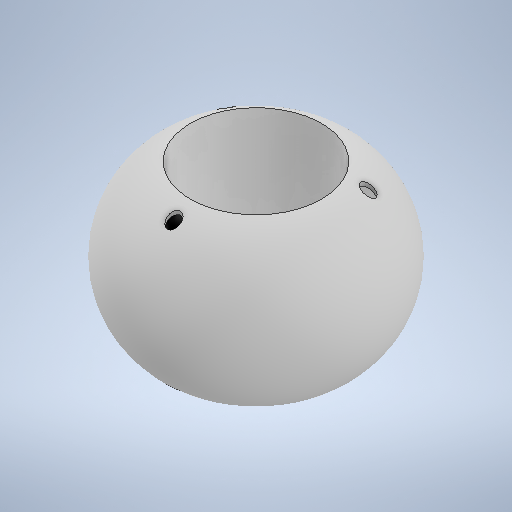
# Autodesk Inventor part: Buoy 5 HalfSphere
Saved by Autodesk Inventor 2025 (Build 290162000, 162)
## iProperties
Created: 2024-06-27
Part Number: Buoy 5 HalfSphere
Material: Generic
Document SubType Name: Modeling
Designer: track
Density: 1 g/cm^3
Appearance: Default
Author: track
Autodesk Inventor part; units mm, degrees
ref_plane "YZ Plane" through (0, 0, 0) normal (1, 0, 0) x (0, 1, 0)
ref_plane "XZ Plane" through (0, 0, 0) normal (0, 1, 0) x (-1, 0, 0)
ref_plane "XY Plane" through (0, 0, 0) normal (0, 0, 1) x (1, 0, 0)
sketch "Sketch1" plane through (0, 0, 0) normal (0, 0, 1) x (1, 0, 0)
  line L0 (0, 0) -> (0, 25.4) construction
  line L1 (30.48, 0) -> (30.48, 76.2)
  line L2 (0, 0) -> (30.48, 0)
  arc A0 (30.48, 0) -> (30.48, 76.2) centre (13.335, 38.1) ccw
  line L3 (31.98, 73.8048) -> (31.98, 2.3952)
  arc A1 (31.98, 2.3952) -> (31.98, 73.8048) centre (13.335, 38.1) ccw
  dimension "d0" = 25.4
  dimension "d1" = 30.48
  dimension "d2" = 76.2
  dimension "d8" = 17.145
  dimension "d9" = 1.5
  constraints: 8 end point, 4 point on circle, 2 centre point, 2 vertical, 1 horizontal, 1 other
  measures "d0" distance of L0.start L0.end
  measures "d1" distance between parallel lines of L1 L0
  measures "d2" distance of L1.start L1.end
  measures "d8" distance from line of A0.centre L1
  measures "d9" radial gap between concentric circles of A0 A1
revolve "Revolution1" add sketch "Sketch1" angle 360 about axis through (0, 0, 0) along (0, 1, 0)
sketch "Sketch2" plane through (0, 0, 0) normal (0, 1, 0) x (-1, 0, 0)
  circle A0 centre (0, 38.1) radius 3
  line L0 (0, 0) -> (0, 38.1) construction
  dimension "d11" = 6
  dimension "d12" = 38.1
  constraints: 2 end point, 1 centre point, 1 vertical
  measures "d11" diameter of A0
  measures "d12" distance of L0.start L0.end
extrude "Extrusion1" cut sketch "Sketch2" along normal blind 76.2
pattern_circular "Circular Pattern1" count 3 over 360 about axis through (0, 38.1, 0) along (0, 1, 0) of "Extrusion1"
body "Solid1"
